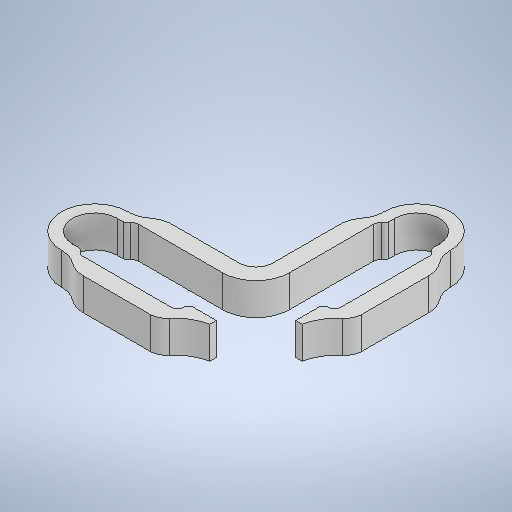
# Autodesk Inventor part: L3 Gearbox CoverUPDATED
Saved by Autodesk Inventor 2025.1 (Build 291241020, 241B)
## iProperties
Created: 2024-09-19
Part Number: L3 Gearbox CoverUPDATED
Material: Generic
Document SubType Name: Modeling
Designer: t205b
Density: 1 g/cm^3
Appearance: Default
Author: t205b
Autodesk Inventor part; units mm, degrees
ref_plane "YZ Plane" through (0, 0, 0) normal (1, 0, 0) x (0, 1, 0)
ref_plane "XZ Plane" through (0, 0, 0) normal (0, 1, 0) x (-1, 0, 0)
ref_plane "XY Plane" through (0, 0, 0) normal (0, 0, 1) x (1, 0, 0)
sketch "Sketch1" plane through (0, 0, 0) normal (0, 1, 0) x (-1, 0, 0)
  line L0 (-25.4, 174.625) -> (-19.05, 174.625)
  line L1 (25.4, 0) -> (25.4, 11.4869)
  line L2 (25.4, 11.4869) -> (31.75, 11.4869)
  line L3 (31.75, 11.4869) -> (31.75, 152.2499)
  line L4 (31.75, 152.2499) -> (172.513, 152.2499)
  line L5 (172.513, 152.2499) -> (172.513, 158.5999)
  line L6 (172.513, 158.5999) -> (183.9999, 158.5999)
  arc A0 (-25.4, 0) -> (25.4, 0) centre (0, 0) ccw
  line L7 (183.9999, 209.3999) -> (172.513, 209.3999)
  line L8 (172.513, 209.3999) -> (172.513, 215.7499)
  line L9 (172.513, 215.7499) -> (58.213, 215.7499)
  line L10 (58.213, 215.7499) -> (58.213, 203.0499)
  line L11 (58.213, 203.0499) -> (9.3749, 203.0499)
  line L12 (9.3749, 203.0499) -> (9.3749, 209.3999)
  line L13 (9.3749, 209.3999) -> (60.1749, 209.3999)
  line L14 (60.1749, 209.3999) -> (60.1749, 234.7999)
  line L15 (60.1749, 234.7999) -> (145.8999, 234.7999)
  arc A1 (183.9999, 158.5999) -> (183.9999, 209.3999) centre (183.9999, 183.9999) ccw
  arc A2 (183.9999, 145.8999) -> (183.9999, 222.0999) centre (183.9999, 183.9999) ccw
  line L16 (145.8999, 133.1999) -> (50.8, 133.1999)
  line L17 (50.8, 133.1999) -> (50.8, 38.1)
  arc A3 (-38.1, 0) -> (38.1, 0) centre (0, 0) ccw
  line L18 (-50.8, 38.1) -> (-50.8, 123.825)
  line L19 (-25.4, 0) -> (-25.4, 11.4869)
  line L20 (-25.4, 11.4869) -> (-31.75, 11.4869)
  line L21 (-31.75, 11.4869) -> (-31.75, 125.7869)
  line L22 (183.9999, 145.8999) -> (164.9499, 145.8999) construction
  line L23 (164.9499, 145.8999) -> (164.9499, 133.1999) construction
  line L24 (164.9499, 133.1999) -> (145.8999, 133.1999) construction
  spline S0 degree 3 poles (183.9999, 145.8999) (164.9499, 145.8999) (164.9499, 133.1999) (145.8999, 133.1999) knots 1 1 1 1 2 2 2 2
  line L25 (38.1, 0) -> (38.1, 19.05) construction
  line L26 (38.1, 19.05) -> (50.8, 19.05) construction
  line L27 (50.8, 19.05) -> (50.8, 38.1) construction
  spline S1 degree 3 poles (38.1, 0) (38.1, 19.05) (50.8, 19.05) (50.8, 38.1) knots 1 1 1 1 2 2 2 2
  line L28 (-38.1, 0) -> (-38.1, 19.05) construction
  line L29 (-38.1, 19.05) -> (-50.8, 19.05) construction
  line L30 (-50.8, 19.05) -> (-50.8, 38.1) construction
  spline S2 degree 3 poles (-38.1, 0) (-38.1, 19.05) (-50.8, 19.05) (-50.8, 38.1) knots 1 1 1 1 2 2 2 2
  line L31 (-31.75, 125.7869) -> (-19.05, 125.7869)
  line L32 (-19.05, 125.7869) -> (-19.05, 174.625)
  line L33 (-50.8, 123.825) -> (-25.4, 123.825)
  line L34 (-25.4, 123.825) -> (-25.4, 174.625)
  line L35 (58.213, 203.0499) -> (70.913, 203.0499)
  line L36 (70.913, 203.0499) -> (70.913, 215.7499)
  line L37 (-31.75, 113.0869) -> (-19.05, 113.0869)
  line L38 (-19.05, 113.0869) -> (-19.05, 125.7869)
  line L39 (183.9999, 222.0999) -> (164.9499, 222.0999) construction
  line L40 (164.9499, 222.0999) -> (164.9499, 234.7999) construction
  line L41 (164.9499, 234.7999) -> (145.8999, 234.7999) construction
  spline S3 degree 3 poles (183.9999, 222.0999) (164.9499, 222.0999) (164.9499, 234.7999) (145.8999, 234.7999) knots 1 1 1 1 2 2 2 2
  dimension "d1" = 38.1
  dimension "d2" = 38.1
  dimension "d3" = 25.4
  dimension "d4" = 25.4
  dimension "d6" = 19.05
  dimension "d7" = 19.05
  dimension "d8" = 19.05
  dimension "d9" = 25.4
  dimension "d10" = 101.6
  dimension "d11" = 101.6
  dimension "d17" = 19.05
  dimension "d18" = 19.05
  dimension "d19" = 12.7
  dimension "d23" = 12.7
  dimension "d24" = 19.05
  dimension "d25" = 19.05
  dimension "d30" = 12.7
  dimension "d33" = 6.35
  dimension "d47" = 19.05
  dimension "d48" = 19.05
  dimension "d49" = 12.7
  dimension "d50" = 12.7
  dimension "d51" = 25.4
  dimension "d52" = 123.825
  dimension "d53" = 133.1999
  dimension "d54" = 133.1999
  dimension "d55" = 11.4869
  dimension "d56" = 11.4869
  dimension "d57" = 50.8
  dimension "d58" = 123.825
  dimension "d59" = 50.8
  dimension "d60" = 114.3
  dimension "d61" = 114.3
  dimension "d62" = 12.7
  dimension "d63" = 12.7
  dimension "d64" = 19.05
  dimension "d65" = 19.05
  dimension "d66" = 12.7
  dimension "d70" = 126.8499
  constraints: 61 end point, 22 perpendicular, 8 horizontal, 8 point on circle, 5 vertical, 4 centre point, 4 tangent, 2 concentric, 2 parallel, 2 point on line, 1 coincident, 1 collinear, 1 horizontal alignment, 1 vertical alignment, 13 other
  measures "d1" radius of A3
  measures "d2" radius of A2
  measures "d3" radius of A0
  measures "d4" radius of A1
  measures "d6" distance between parallel lines of L3 L17
  measures "d7" distance between parallel lines of L4 L16
  measures "d8" distance between parallel lines of L15 L9
  measures "d9" distance of L13.end L14.end
  measures "d10" distance between parallel lines of L16 L15
  measures "d11" distance between parallel lines of L18 L17
  measures "d17" distance of L23.end L16.start
  measures "d18" distance of L22.start L22.end
  measures "d19" distance of L22.end L23.end
  measures "d23" distance of L25.end L26.end
  measures "d24" distance of L26.end L17.end
  measures "d25" distance of L25.start L25.end
  measures "d30" distance of L9.end L10.end
  measures "d33" distance of L19.end L20.end
  measures "d47" distance of L28.start L28.end
  measures "d48" distance of L29.end L18.start
  measures "d49" distance of L28.end L29.end
  measures "d50" distance of L21.end L31.end
  measures "d51" distance of L18.end L33.end
  measures "d52" vertical distance of L18.end A0.centre
  measures "d53" distance from line of L16 A0.centre
  measures "d54" distance from line of A1.centre L17
  measures "d55" distance from line of A1.centre L8
  measures "d56" distance from line of L2 A3.centre
  measures "d57" distance of L12.end L13.end
  measures "d58" distance from line of L14 A1.centre
  measures "d59" distance of L33.end L0.start
  measures "d60" distance between parallel lines of L10 L8
  measures "d61" distance between parallel lines of L31 L20
  measures "d62" distance of L37.end L31.end
  measures "d63" distance between parallel lines of L36 L10
  measures "d64" distance of L40.end L15.end
  measures "d65" distance of L39.start L39.end
  measures "d66" distance of L39.end L40.end
  measures "d70" distance between parallel lines of L26 L22
extrude "Extrusion1" add sketch "Sketch1" along normal blind 34.417 contours L0 L32 L31 L34 | L31 L38 L37 L21 L33 L34 | L21 L20 L19 A0 L1 L2 L3 L4 L5 L6 A1 L7 L8 L9 L14 L15 S3 A2 S0 L16 L17 S1 A3 S2 L18 L33 | L9 L36 L35 L10 L13 L14 | L10 L11 L12 L13
fillet "Fillet1" radius 50.8 2 edges at (-60.1749, 17.2085, 209.3999) (25.4, 17.2085, 123.825)
fillet "Fillet2" radius 19.05 3 edges at (50.8, 17.2085, 123.825) (-60.1749, 17.2085, 234.7999) (-50.8, 17.2085, 133.1999)
fillet "Fillet4" radius 38.1 1 edges at (-31.75, 17.2085, 152.2499)
extrude "Extrusion2" cut sketch "Sketch1" along normal blind 34.417 contours L34 L33 L21 L31 | L31 L38 L37 L21 L33 L34 | L14 L13 L10 L9 | L9 L36 L35 L10 L13 L14
fillet "Fillet5" radius 6.35 12 edges at (-172.513, 17.2085, 215.7499) (-172.513, 17.2085, 209.3999) (-58.213, 17.2085, 215.7499) (-58.213, 17.2085, 203.0499) (31.75, 17.2085, 125.7869) (19.05, 17.2085, 125.7869) (31.75, 17.2085, 11.4869) (25.4, 17.2085, 11.4869) (-25.4, 17.2085, 11.4869) (-31.75, 17.2085, 11.4869) (-172.513, 17.2085, 152.2499) (-172.513, 17.2085, 158.5999)
sketch "Sketch2" plane through (0, 34.417, 0) normal (0, 1, 0) x (1, 0, 0)
  circle A0 centre (38.1, -111.125) radius 2.65
  circle A1 centre (38.1, -85.725) radius 2.65
  circle A2 centre (38.1, -60.325) radius 2.65
  circle A3 centre (38.1, -34.925) radius 2.65
  circle A4 centre (31.75, 0) radius 2.65
  circle A5 centre (-31.75, 0) radius 2.65
  circle A6 centre (-38.1, -34.925) radius 2.65
  circle A7 centre (-38.1, -60.325) radius 2.65
  circle A8 centre (-38.1, -85.725) radius 2.65
  circle A9 centre (-38.1, -111.125) radius 2.65
  circle A10 centre (-72.8749, -145.8999) radius 2.65
  circle A11 centre (-98.2749, -145.8999) radius 2.65
  circle A12 centre (-123.6749, -145.8999) radius 2.65
  circle A13 centre (-149.0749, -145.8999) radius 2.65
  circle A14 centre (-183.9999, -152.2499) radius 2.65
  circle A15 centre (-98.2749, -222.0999) radius 2.65
  circle A16 centre (-72.8749, -222.0999) radius 2.65
  circle A17 centre (-123.6749, -222.0999) radius 2.65
  circle A18 centre (-183.9999, -215.7499) radius 2.65
  circle A19 centre (-149.0749, -222.0999) radius 2.65
  arc A20 (-177.1615, -158.5999) -> (-171.6623, -155.4249) centre (-177.1615, -152.2499) ccw projected
  arc A21 (-166.163, -152.2499) -> (-171.6623, -155.4249) centre (-166.163, -158.5999) ccw projected
  line L0 (-166.163, -152.2499) -> (-69.85, -152.2499) projected
  arc A22 (-69.85, -152.2499) -> (-31.75, -114.1499) centre (-69.85, -114.1499) ccw projected
  line L1 (-31.75, -114.1499) -> (-31.75, -17.8369) projected
  arc A23 (-28.575, -12.3376) -> (-31.75, -17.8369) centre (-25.4, -17.8369) ccw projected
  arc A24 (-28.575, -12.3376) -> (-25.4, -6.8384) centre (-31.75, -6.8384) ccw projected
  line L2 (-25.4, -6.8384) -> (-25.4, 0) projected
  arc A25 (25.4, 0) -> (-25.4, 0) centre (0, 0) ccw projected
  line L3 (25.4, 0) -> (25.4, -6.8384) projected
  arc A26 (25.4, -6.8384) -> (28.575, -12.3376) centre (31.75, -6.8384) ccw projected
  arc A27 (31.75, -17.8369) -> (28.575, -12.3376) centre (25.4, -17.8369) ccw projected
  line L4 (31.75, -17.8369) -> (31.75, -119.4369) projected
  arc A28 (25.4, -125.7869) -> (31.75, -119.4369) centre (25.4, -119.4369) ccw projected
  arc A29 (25.4, -125.7869) -> (19.05, -132.1369) centre (25.4, -132.1369) ccw projected
  line L5 (19.05, -132.1369) -> (19.05, -174.625) projected
  line L6 (19.05, -174.625) -> (25.4, -174.625) projected
  line L7 (25.4, -174.625) -> (25.4, -167.8191) projected
  arc A30 (43.8727, -128.6325) -> (25.4, -167.8191) centre (76.2, -167.8191) ccw projected
  arc A31 (43.8727, -128.6325) -> (50.8, -113.9376) centre (31.75, -113.9376) ccw projected
  line L8 (50.8, -113.9376) -> (50.8, -38.1) projected
  arc A32 (38.1, 0) -> (-38.1, 0) centre (0, 0) ccw projected
  line L9 (-50.8, -38.1) -> (-50.8, -114.1499) projected
  arc A33 (-69.85, -133.1999) -> (-50.8, -114.1499) centre (-69.85, -114.1499) ccw projected
  line L10 (-69.85, -133.1999) -> (-145.8999, -133.1999) projected
  arc A34 (-183.9999, -145.8999) -> (-183.9999, -222.0999) centre (-183.9999, -183.9999) ccw projected
  line L11 (-145.8999, -234.7999) -> (-70.0623, -234.7999) projected
  arc A35 (-70.0623, -234.7999) -> (-55.3674, -227.8726) centre (-70.0623, -215.7499) ccw projected
  arc A36 (-16.1808, -209.3999) -> (-55.3674, -227.8726) centre (-16.1808, -260.1999) ccw projected
  line L12 (-16.1808, -209.3999) -> (-9.3749, -209.3999) projected
  line L13 (-9.3749, -209.3999) -> (-9.3749, -203.0499) projected
  line L14 (-9.3749, -203.0499) -> (-51.863, -203.0499) projected
  arc A37 (-51.863, -203.0499) -> (-58.213, -209.3999) centre (-51.863, -209.3999) ccw projected
  arc A38 (-64.563, -215.7499) -> (-58.213, -209.3999) centre (-64.563, -209.3999) ccw projected
  line L15 (-64.563, -215.7499) -> (-166.163, -215.7499) projected
  arc A39 (-171.6623, -212.5749) -> (-166.163, -215.7499) centre (-166.163, -209.3999) ccw projected
  arc A40 (-171.6623, -212.5749) -> (-177.1615, -209.3999) centre (-177.1615, -215.7499) ccw projected
  line L16 (-177.1615, -209.3999) -> (-183.9999, -209.3999) projected
  arc A41 (-183.9999, -158.5999) -> (-183.9999, -209.3999) centre (-183.9999, -183.9999) ccw projected
  line L17 (-183.9999, -158.5999) -> (-177.1615, -158.5999) projected
  dimension "d80" = 5.3
  dimension "d81" = 25.4
  dimension "d82" = 25.4
  dimension "d83" = 25.4
  dimension "d84" = 25.4
  dimension "d85" = 25.4
  dimension "d86" = 25.4
  dimension "d87" = 25.4
  dimension "d88" = 25.4
  dimension "d89" = 25.4
  dimension "d90" = 25.4
  dimension "d91" = 25.4
  dimension "d92" = 25.4
  dimension "d93" = 31.75
  dimension "d94" = 31.75
  dimension "d95" = 31.75
  dimension "d96" = 31.75
  dimension "d97" = 76.2
  dimension "d98" = 38.1
  dimension "d99" = 76.2
  dimension "d100" = 38.1
  dimension "d101" = 34.925
  dimension "d102" = 34.925
  dimension "d103" = 34.925
  dimension "d104" = 34.925
  constraints: 20 centre point, 19 equal radius, 8 horizontal alignment, 8 vertical alignment, 4 other
  measures "d80" diameter of A0
  measures "d81" distance of A1.centre A0.centre
  measures "d82" distance of A2.centre A1.centre
  measures "d83" distance of A3.centre A2.centre
  measures "d84" distance of A7.centre A6.centre
  measures "d85" distance of A8.centre A7.centre
  measures "d86" distance of A9.centre A8.centre
  measures "d87" distance of A11.centre A10.centre
  measures "d88" distance of A11.centre A12.centre
  measures "d89" distance of A12.centre A13.centre
  measures "d90" distance of A15.centre A16.centre
  measures "d91" distance of A17.centre A15.centre
  measures "d92" distance of A17.centre A19.centre
  measures "d93" distance of A4.centre point (0, 0)
  measures "d94" distance of point (0, 0) A5.centre
  measures "d95" distance of A34.centre A18.centre
  measures "d96" distance of A14.centre A34.centre
  measures "d97" distance of A6.centre A3.centre
  measures "d98" horizontal distance of point (0, 0) A6.centre
  measures "d99" distance of A19.centre A13.centre
  measures "d100" vertical distance of A34.centre A19.centre
  measures "d101" vertical distance of A4.centre A3.centre
  measures "d102" vertical distance of A5.centre A6.centre
  measures "d103" horizontal distance of A13.centre A14.centre
  measures "d104" horizontal distance of A19.centre A18.centre
extrude "Extrusion3" cut sketch "Sketch2" against normal through all
sketch "Sketch3" plane through (0, 34.417, 0) normal (0, 1, 0) x (1, 0, 0)
  circle A0 centre (38.1, -60.325) radius 2.65 projected
  circle A1 centre (-38.1, -34.925) radius 2.65 projected
  circle A2 centre (-72.8749, -145.8999) radius 2.65 projected
  circle A3 centre (-149.0749, -145.8999) radius 2.65 projected
  circle A4 centre (-183.9999, -215.7499) radius 2.65 projected
  circle A5 centre (-123.6749, -222.0999) radius 2.65 projected
  circle A6 centre (-123.6749, -145.8999) radius 2.65 projected
  circle A7 centre (-38.1, -111.125) radius 2.65 projected
  circle A8 centre (-31.75, 0) radius 2.65 projected
  circle A9 centre (38.1, -85.725) radius 2.65 projected
  circle A10 centre (38.1, -34.925) radius 2.65 projected
  circle A11 centre (-38.1, -60.325) radius 2.65 projected
  circle A12 centre (-72.8749, -222.0999) radius 2.65 projected
  circle A13 centre (-183.9999, -152.2499) radius 2.65 projected
  circle A14 centre (-149.0749, -222.0999) radius 2.65 projected
  circle A15 centre (-98.2749, -222.0999) radius 2.65 projected
  circle A16 centre (-98.2749, -145.8999) radius 2.65 projected
  circle A17 centre (-38.1, -85.725) radius 2.65 projected
  circle A18 centre (31.75, 0) radius 2.65 projected
  circle A19 centre (38.1, -111.125) radius 2.65 projected
  arc A20 (-177.1615, -158.5999) -> (-171.6623, -155.4249) centre (-177.1615, -152.2499) ccw projected
  arc A21 (-166.163, -152.2499) -> (-171.6623, -155.4249) centre (-166.163, -158.5999) ccw projected
  line L0 (-166.163, -152.2499) -> (-69.85, -152.2499) projected
  arc A22 (-69.85, -152.2499) -> (-31.75, -114.1499) centre (-69.85, -114.1499) ccw projected
  line L1 (-31.75, -114.1499) -> (-31.75, -17.8369) projected
  arc A23 (-28.575, -12.3376) -> (-31.75, -17.8369) centre (-25.4, -17.8369) ccw projected
  arc A24 (-28.575, -12.3376) -> (-25.4, -6.8384) centre (-31.75, -6.8384) ccw projected
  line L2 (-25.4, -6.8384) -> (-25.4, 0) projected
  arc A25 (25.4, 0) -> (-25.4, 0) centre (0, 0) ccw projected
  line L3 (25.4, 0) -> (25.4, -6.8384) projected
  arc A26 (25.4, -6.8384) -> (28.575, -12.3376) centre (31.75, -6.8384) ccw projected
  arc A27 (31.75, -17.8369) -> (28.575, -12.3376) centre (25.4, -17.8369) ccw projected
  line L4 (31.75, -17.8369) -> (31.75, -119.4369) projected
  arc A28 (25.4, -125.7869) -> (31.75, -119.4369) centre (25.4, -119.4369) ccw projected
  arc A29 (25.4, -125.7869) -> (19.05, -132.1369) centre (25.4, -132.1369) ccw projected
  line L5 (19.05, -132.1369) -> (19.05, -174.625) projected
  line L6 (19.05, -174.625) -> (25.4, -174.625) projected
  line L7 (25.4, -174.625) -> (25.4, -167.8191) projected
  arc A30 (43.8727, -128.6325) -> (25.4, -167.8191) centre (76.2, -167.8191) ccw projected
  arc A31 (43.8727, -128.6325) -> (50.8, -113.9376) centre (31.75, -113.9376) ccw projected
  line L8 (50.8, -113.9376) -> (50.8, -38.1) projected
  arc A32 (38.1, 0) -> (-38.1, 0) centre (0, 0) ccw projected
  line L9 (-50.8, -38.1) -> (-50.8, -114.1499) projected
  arc A33 (-69.85, -133.1999) -> (-50.8, -114.1499) centre (-69.85, -114.1499) ccw projected
  line L10 (-69.85, -133.1999) -> (-145.8999, -133.1999) projected
  arc A34 (-183.9999, -145.8999) -> (-183.9999, -222.0999) centre (-183.9999, -183.9999) ccw projected
  line L11 (-145.8999, -234.7999) -> (-70.0623, -234.7999) projected
  arc A35 (-70.0623, -234.7999) -> (-55.3674, -227.8726) centre (-70.0623, -215.7499) ccw projected
  arc A36 (-16.1808, -209.3999) -> (-55.3674, -227.8726) centre (-16.1808, -260.1999) ccw projected
  line L12 (-16.1808, -209.3999) -> (-9.3749, -209.3999) projected
  line L13 (-9.3749, -209.3999) -> (-9.3749, -203.0499) projected
  line L14 (-9.3749, -203.0499) -> (-51.863, -203.0499) projected
  arc A37 (-51.863, -203.0499) -> (-58.213, -209.3999) centre (-51.863, -209.3999) ccw projected
  arc A38 (-64.563, -215.7499) -> (-58.213, -209.3999) centre (-64.563, -209.3999) ccw projected
  line L15 (-64.563, -215.7499) -> (-166.163, -215.7499) projected
  arc A39 (-171.6623, -212.5749) -> (-166.163, -215.7499) centre (-166.163, -209.3999) ccw projected
  arc A40 (-171.6623, -212.5749) -> (-177.1615, -209.3999) centre (-177.1615, -215.7499) ccw projected
  line L16 (-177.1615, -209.3999) -> (-183.9999, -209.3999) projected
  arc A41 (-183.9999, -158.5999) -> (-183.9999, -209.3999) centre (-183.9999, -183.9999) ccw projected
  line L17 (-183.9999, -158.5999) -> (-177.1615, -158.5999) projected
  arc A42 (43.8727, -128.6325) -> (25.4, -167.8191) centre (76.2, -167.8191) ccw projected
  line L18 (26.4081, -157.7492) -> (19.05, -157.7492)
  line L19 (-26.2506, -203.0499) -> (-26.2506, -210.4079)
  dimension "d108" = 31.9623
  dimension "d109" = 31.9623
  constraints: 4 end point, 2 perpendicular, 2 point on circle, 2 point on line, 4 other
  measures "d108" distance from line of L18 A28.start
  measures "d109" distance from line of L19 A37.end
extrude "Extrusion4" cut sketch "Sketch3" against normal through all contours L18 A30 L7 L6 L5 | A36 L19 L14 L13 L12
sketch "Sketch4" plane through (0, 34.417, 0) normal (0, 1, 0) x (1, 0, 0)
  circle A0 centre (38.1, -111.125) radius 2.65 projected
  circle A1 centre (31.75, 0) radius 2.65 projected
  circle A2 centre (-38.1, -85.725) radius 2.65 projected
  circle A3 centre (-98.2749, -145.8999) radius 2.65 projected
  circle A4 centre (-98.2749, -222.0999) radius 2.65 projected
  circle A5 centre (-149.0749, -222.0999) radius 2.65 projected
  circle A6 centre (-183.9999, -152.2499) radius 2.65 projected
  circle A7 centre (-72.8749, -222.0999) radius 2.65 projected
  circle A8 centre (-38.1, -60.325) radius 2.65 projected
  circle A9 centre (38.1, -34.925) radius 2.65 projected
  circle A10 centre (38.1, -85.725) radius 2.65 projected
  circle A11 centre (-31.75, 0) radius 2.65 projected
  circle A12 centre (-38.1, -111.125) radius 2.65 projected
  circle A13 centre (-123.6749, -145.8999) radius 2.65 projected
  circle A14 centre (-123.6749, -222.0999) radius 2.65 projected
  circle A15 centre (-183.9999, -215.7499) radius 2.65 projected
  circle A16 centre (-149.0749, -145.8999) radius 2.65 projected
  circle A17 centre (-72.8749, -145.8999) radius 2.65 projected
  circle A18 centre (-38.1, -34.925) radius 2.65 projected
  circle A19 centre (38.1, -60.325) radius 2.65 projected
  line L0 (-26.2506, -210.4079) -> (-26.2506, -203.0499) projected
  line L1 (-26.2506, -203.0499) -> (-51.863, -203.0499) projected
  arc A20 (-51.863, -203.0499) -> (-58.213, -209.3999) centre (-51.863, -209.3999) ccw projected
  arc A21 (-64.563, -215.7499) -> (-58.213, -209.3999) centre (-64.563, -209.3999) ccw projected
  line L2 (-64.563, -215.7499) -> (-166.163, -215.7499) projected
  arc A22 (-171.6623, -212.5749) -> (-166.163, -215.7499) centre (-166.163, -209.3999) ccw projected
  arc A23 (-171.6623, -212.5749) -> (-177.1615, -209.3999) centre (-177.1615, -215.7499) ccw projected
  line L3 (-177.1615, -209.3999) -> (-183.9999, -209.3999) projected
  arc A24 (-183.9999, -158.5999) -> (-183.9999, -209.3999) centre (-183.9999, -183.9999) ccw projected
  line L4 (-183.9999, -158.5999) -> (-177.1615, -158.5999) projected
  arc A25 (-177.1615, -158.5999) -> (-171.6623, -155.4249) centre (-177.1615, -152.2499) ccw projected
  arc A26 (-166.163, -152.2499) -> (-171.6623, -155.4249) centre (-166.163, -158.5999) ccw projected
  line L5 (-166.163, -152.2499) -> (-69.85, -152.2499) projected
  arc A27 (-69.85, -152.2499) -> (-31.75, -114.1499) centre (-69.85, -114.1499) ccw projected
  line L6 (-31.75, -114.1499) -> (-31.75, -17.8369) projected
  arc A28 (-28.575, -12.3376) -> (-31.75, -17.8369) centre (-25.4, -17.8369) ccw projected
  arc A29 (-28.575, -12.3376) -> (-25.4, -6.8384) centre (-31.75, -6.8384) ccw projected
  line L7 (-25.4, -6.8384) -> (-25.4, 0) projected
  arc A30 (25.4, 0) -> (-25.4, 0) centre (0, 0) ccw projected
  line L8 (25.4, 0) -> (25.4, -6.8384) projected
  arc A31 (25.4, -6.8384) -> (28.575, -12.3376) centre (31.75, -6.8384) ccw projected
  arc A32 (31.75, -17.8369) -> (28.575, -12.3376) centre (25.4, -17.8369) ccw projected
  line L9 (31.75, -17.8369) -> (31.75, -119.4369) projected
  arc A33 (25.4, -125.7869) -> (31.75, -119.4369) centre (25.4, -119.4369) ccw projected
  arc A34 (25.4, -125.7869) -> (19.05, -132.1369) centre (25.4, -132.1369) ccw projected
  line L10 (19.05, -132.1369) -> (19.05, -157.7492) projected
  line L11 (19.05, -157.7492) -> (26.4081, -157.7492) projected
  arc A35 (43.8727, -128.6325) -> (26.4081, -157.7492) centre (76.2, -167.8191) ccw projected
  arc A36 (43.8727, -128.6325) -> (50.8, -113.9376) centre (31.75, -113.9376) ccw projected
  line L12 (50.8, -113.9376) -> (50.8, -38.1) projected
  spline S0 degree 3 poles (50.8, -38.1) (50.8, -19.05) (38.1, -19.05) (38.1, 0) knots 0 0 0 0 1 1 1 1 projected
  arc A37 (38.1, 0) -> (-38.1, 0) centre (0, 0) ccw projected
  spline S1 degree 3 poles (-38.1, 0) (-38.1, -19.05) (-50.8, -19.05) (-50.8, -38.1) knots 0 0 0 0 1 1 1 1 projected
  line L13 (-50.8, -38.1) -> (-50.8, -114.1499) projected
  arc A38 (-69.85, -133.1999) -> (-50.8, -114.1499) centre (-69.85, -114.1499) ccw projected
  line L14 (-69.85, -133.1999) -> (-145.8999, -133.1999) projected
  spline S2 degree 3 poles (-145.8999, -133.1999) (-164.9499, -133.1999) (-164.9499, -145.8999) (-183.9999, -145.8999) knots 0 0 0 0 1 1 1 1 projected
  arc A39 (-183.9999, -145.8999) -> (-183.9999, -222.0999) centre (-183.9999, -183.9999) ccw projected
  spline S3 degree 3 poles (-183.9999, -222.0999) (-164.9499, -222.0999) (-164.9499, -234.7999) (-145.8999, -234.7999) knots 0 0 0 0 1 1 1 1 projected
  line L15 (-145.8999, -234.7999) -> (-70.0623, -234.7999) projected
  arc A40 (-70.0623, -234.7999) -> (-55.3674, -227.8726) centre (-70.0623, -215.7499) ccw projected
  arc A41 (-26.2506, -210.4079) -> (-55.3674, -227.8726) centre (-16.1808, -260.1999) ccw projected
  constraints: 4 other
extrude "Extrusion5" add sketch "Sketch4" along normal blind 0.635
sketch "Sketch5" plane through (0, 35.052, 0) normal (0, 1, 0) x (1, 0, 0)
  spline S0 degree 3 poles (-145.8999, -133.1999) (-164.9499, -133.1999) (-164.9499, -145.8999) (-183.9999, -145.8999) knots 0 0 0 0 1 1 1 1 projected
  arc A0 (-183.9999, -145.8999) -> (-183.9999, -222.0999) centre (-183.9999, -183.9999) ccw projected
  spline S1 degree 3 poles (-183.9999, -222.0999) (-164.9499, -222.0999) (-164.9499, -234.7999) (-145.8999, -234.7999) knots 0 0 0 0 1 1 1 1 projected
  line L0 (-145.8999, -234.7999) -> (-70.0623, -234.7999) projected
  arc A1 (-70.0623, -234.7999) -> (-55.3674, -227.8726) centre (-70.0623, -215.7499) ccw projected
  arc A2 (-26.2506, -210.4079) -> (-55.3674, -227.8726) centre (-16.1808, -260.1999) ccw projected
  line L1 (-26.2506, -210.4079) -> (-26.2506, -203.0499) projected
  line L2 (-26.2506, -203.0499) -> (-51.863, -203.0499) projected
  arc A3 (-51.863, -203.0499) -> (-58.213, -209.3999) centre (-51.863, -209.3999) ccw projected
  arc A4 (-64.563, -215.7499) -> (-58.213, -209.3999) centre (-64.563, -209.3999) ccw projected
  line L3 (-64.563, -215.7499) -> (-166.163, -215.7499) projected
  arc A5 (-171.6623, -212.5749) -> (-166.163, -215.7499) centre (-166.163, -209.3999) ccw projected
  arc A6 (-171.6623, -212.5749) -> (-177.1615, -209.3999) centre (-177.1615, -215.7499) ccw projected
  line L4 (-177.1615, -209.3999) -> (-183.9999, -209.3999) projected
  arc A7 (-183.9999, -158.5999) -> (-183.9999, -209.3999) centre (-183.9999, -183.9999) ccw projected
  line L5 (-183.9999, -158.5999) -> (-177.1615, -158.5999) projected
  arc A8 (-177.1615, -158.5999) -> (-171.6623, -155.4249) centre (-177.1615, -152.2499) ccw projected
  arc A9 (-166.163, -152.2499) -> (-171.6623, -155.4249) centre (-166.163, -158.5999) ccw projected
  line L6 (-166.163, -152.2499) -> (-69.85, -152.2499) projected
  arc A10 (-69.85, -152.2499) -> (-31.75, -114.1499) centre (-69.85, -114.1499) ccw projected
  line L7 (-31.75, -114.1499) -> (-31.75, -17.8369) projected
  arc A11 (-28.575, -12.3376) -> (-31.75, -17.8369) centre (-25.4, -17.8369) ccw projected
  arc A12 (-28.575, -12.3376) -> (-25.4, -6.8384) centre (-31.75, -6.8384) ccw projected
  line L8 (-25.4, -6.8384) -> (-25.4, 0) projected
  arc A13 (25.4, 0) -> (-25.4, 0) centre (0, 0) ccw projected
  line L9 (25.4, 0) -> (25.4, -6.8384) projected
  arc A14 (25.4, -6.8384) -> (28.575, -12.3376) centre (31.75, -6.8384) ccw projected
  arc A15 (31.75, -17.8369) -> (28.575, -12.3376) centre (25.4, -17.8369) ccw projected
  line L10 (31.75, -17.8369) -> (31.75, -119.4369) projected
  arc A16 (25.4, -125.7869) -> (31.75, -119.4369) centre (25.4, -119.4369) ccw projected
  arc A17 (25.4, -125.7869) -> (19.05, -132.1369) centre (25.4, -132.1369) ccw projected
  line L11 (19.05, -132.1369) -> (19.05, -157.7492) projected
  line L12 (19.05, -157.7492) -> (26.4081, -157.7492) projected
  arc A18 (43.8727, -128.6325) -> (26.4081, -157.7492) centre (76.2, -167.8191) ccw projected
  arc A19 (43.8727, -128.6325) -> (50.8, -113.9376) centre (31.75, -113.9376) ccw projected
  line L13 (50.8, -113.9376) -> (50.8, -38.1) projected
  spline S2 degree 3 poles (50.8, -38.1) (50.8, -19.05) (38.1, -19.05) (38.1, 0) knots 0 0 0 0 1 1 1 1 projected
  arc A20 (38.1, 0) -> (-38.1, 0) centre (0, 0) ccw projected
  spline S3 degree 3 poles (-38.1, 0) (-38.1, -19.05) (-50.8, -19.05) (-50.8, -38.1) knots 0 0 0 0 1 1 1 1 projected
  line L14 (-50.8, -38.1) -> (-50.8, -114.1499) projected
  arc A21 (-69.85, -133.1999) -> (-50.8, -114.1499) centre (-69.85, -114.1499) ccw projected
  line L15 (-69.85, -133.1999) -> (-145.8999, -133.1999) projected
  circle A22 centre (38.1, -60.325) radius 2.65 projected
  circle A23 centre (-123.6749, -222.0999) radius 2.65 projected
  circle A24 centre (-38.1, -111.125) radius 2.65 projected
  circle A25 centre (38.1, -85.725) radius 2.65 projected
  circle A26 centre (-38.1, -60.325) radius 2.65 projected
  circle A27 centre (-72.8749, -222.0999) radius 2.65 projected
  circle A28 centre (-98.2749, -222.0999) radius 2.65 projected
  circle A29 centre (-98.2749, -145.8999) radius 2.65 projected
  circle A30 centre (-38.1, -85.725) radius 2.65 projected
  circle A31 centre (38.1, -111.125) radius 2.65 projected
  circle A32 centre (-123.6749, -145.8999) radius 2.65 projected
  circle A33 centre (-72.8749, -145.8999) radius 2.65 projected
  circle A34 centre (-38.1, -34.925) radius 2.65 projected
  circle A35 centre (-149.0749, -145.8999) radius 2.65 projected
  circle A36 centre (-183.9999, -215.7499) radius 2.65 projected
  circle A37 centre (-31.75, 0) radius 2.65 projected
  circle A38 centre (38.1, -34.925) radius 2.65 projected
  circle A39 centre (-183.9999, -152.2499) radius 2.65 projected
  circle A40 centre (-149.0749, -222.0999) radius 2.65 projected
  circle A41 centre (31.75, 0) radius 2.65 projected
  constraints: 4 other
extrude "Extrusion6" add sketch "Sketch5" along normal blind 1.524 contours L15 A21 L14 S3 A20 S2 L13 A19 A18 L12 L11 A17 A16 L10 A15 A14 L9 A13 L8 A12 A11 L7 A10 L6 A9 A8 L5 A7 L4 A6 A5 L3 A4 A3 L2 L1 A2 A1 L0 S1 A0 S0 | A22 | A23 | A24 | A25 | A26 | A27 | A28 | A29 | A30 | A31 | A32 | A33 | A34 | A35 | A36 | A37 | A38 | A39 | A40 | A41
body "Solid1"
